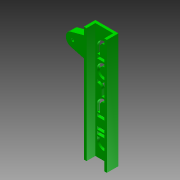
# Autodesk Inventor part: TabletMount-Mast-Left
Saved by Autodesk Inventor 2012 (Build 160160000, 160)
## iProperties
Created: 2013-10-06
Part Number: TabletMount-Mast-Left
Material: Default
Document SubType Name: Modeling
Designer: joe_000
Density: 1 g/cm^3
Author: joe_000
Autodesk Inventor part; units mm, degrees
ref_plane "YZ Plane" through (0, 0, 0) normal (1, 0, 0) x (0, 1, 0)
ref_plane "XZ Plane" through (0, 0, 0) normal (0, 1, 0) x (-1, 0, 0)
ref_plane "XY Plane" through (0, 0, 0) normal (0, 0, 1) x (1, 0, 0)
sketch "Sketch1" plane through (0, 0, 0) normal (0, 1, 0) x (-1, 0, 0)
  line L0 (0, 12.7) -> (0, 0)
  line L1 (0, 0) -> (25.4, 0)
  line L2 (25.4, 0) -> (25.4, 12.7)
  line L3 (25.4, 12.7) -> (22.479, 12.7)
  line L4 (22.479, 12.7) -> (22.479, 2.921)
  line L5 (22.479, 2.921) -> (2.921, 2.921)
  line L6 (2.921, 2.921) -> (2.921, 12.7)
  line L7 (2.921, 12.7) -> (0, 12.7)
  dimension "d0" = 19.558
  dimension "d1" = 2.921
  dimension "d2" = 2.921
  dimension "d3" = 2.921
  dimension "d4" = 9.779
  constraints: 16 end point, 5 parallel, 1 collinear, 1 horizontal, 1 perpendicular, 1 vertical
  measures "d0" distance of L4.end L5.end
  measures "d1" distance between parallel lines of L0 L6
  measures "d2" distance between parallel lines of L2 L4
  measures "d3" distance between parallel lines of L1 L5
  measures "d4" distance between parallel lines of L5 L3
extrude "Extrusion1" add sketch "Sketch1" along normal blind 127
sketch "Sketch3" plane through (0, 0, 0) normal (0, 0, -1) x (-1, 0, 0)
  line L0 (0, 0) -> (0, 127) projected
  line L1 (25.4, 0) -> (25.4, 127) projected
  line L2 (25.4, 115.4147) -> (44.45, 110.3102)
  line L3 (25.4, 90.8361) -> (44.45, 95.9406)
  arc A0 (44.45, 95.9406) -> (44.45, 110.3102) centre (42.5248, 103.1254) ccw
  point P0 (0, 115.8525)
  point P1 (0, 86.0657)
  dimension "d9" = 75
  dimension "d10" = 75
  dimension "d11" = 19.05
  dimension "d12" = 19.05
  constraints: 4 end point, 4 point on line, 2 point on circle, 1 centre point, 1 tangent
  measures "d9" angle of L1 L2
  measures "d10" angle of L1 L3
  measures "d11" horizontal distance of L2.start L2.end
  measures "d12" horizontal distance of L3.start L3.end
extrude "Extrusion2" add sketch "Sketch3" against normal blind 8.0433
hole "Hole1" at (-42.5248, 103.1254, 0) direction (0, 0, 1) diameter 3 end through all
fillet "Fillet1" radius 3.175 2 edges at (-25.4, 115.4147, 4.0217) (-25.4, 90.8361, 4.0217)
sketch "Sketch4" plane through (0, 0, 0) normal (0, 0, -1) x (-1, 0, 0)
  line L0 (5.2487, 9.5266) -> (5.2487, 115.9417) construction
  line L1 (5.2487, 115.9417) -> (20.5107, 115.9417) construction
  line L2 (20.5107, 115.9417) -> (20.5107, 9.5266) construction
  line L3 (20.5107, 9.5266) -> (5.2487, 9.5266) construction
  line L4 (5.2487, 17.8252) -> (5.2487, 24.8769)
  line L5 (5.2487, 24.8769) -> (20.5107, 24.8769)
  line L6 (20.5107, 24.8769) -> (20.5107, 21.8201)
  line L7 (20.5107, 21.8201) -> (8.2172, 21.8201)
  line L8 (8.2172, 21.8201) -> (8.2283, 19.0833)
  line L9 (8.2283, 19.0833) -> (8.2283, 18.4322)
  spline S0 degree 2 poles (8.2283, 18.4322) (8.2283, 16.1479) (8.4159, 15.894) knots 0 0 0 1 1 1
  spline S1 degree 2 poles (8.4159, 15.894) (8.7911, 14.5256) (9.9939, 13.5766) knots 0 0 0 1 1 1
  spline S2 degree 2 poles (9.9939, 13.5766) (11.4506, 12.5613) (12.8852, 12.5613) knots 0 0 0 1 1 1
  spline S3 degree 2 poles (12.8852, 12.5613) (14.673, 12.5613) (16.1628, 13.9408) knots 0 0 0 1 1 1
  spline S4 degree 2 poles (16.1628, 13.9408) (17.0346, 14.8677) (17.2222, 15.5299) knots 0 0 0 1 1 1
  spline S5 degree 2 poles (17.2222, 15.5299) (17.5532, 16.192) (17.5532, 17.8252) knots 0 0 0 1 1 1
  line L10 (17.5532, 17.8252) -> (17.5532, 19.9551)
  line L11 (17.5532, 19.9551) -> (20.5107, 19.9551)
  line L12 (20.5107, 19.9551) -> (20.5107, 17.4059)
  spline S6 degree 2 poles (20.5107, 17.4059) (20.5107, 14.5698) (19.021, 12.6055) knots 0 0 0 1 1 1
  spline S7 degree 2 poles (19.021, 12.6055) (17.8953, 11.1929) (16.9904, 10.7074) knots 0 0 0 1 1 1
  spline S8 degree 2 poles (16.9904, 10.7074) (15.1034, 9.5266) (13.128, 9.5266) knots 0 0 0 1 1 1
  line L13 (13.128, 9.5266) -> (12.6866, 9.5266)
  spline S9 degree 2 poles (12.6866, 9.5266) (9.9388, 9.5266) (7.6323, 11.5902) knots 0 0 0 1 1 1
  spline S10 degree 2 poles (7.6323, 11.5902) (6.4184, 12.8372) (6.0984, 13.6318) knots 0 0 0 1 1 1
  spline S11 degree 2 poles (6.0984, 13.6318) (5.7894, 14.2056) (5.5025, 15.2098) knots 0 0 0 1 1 1
  spline S12 degree 2 poles (5.5025, 15.2098) (5.2487, 16.1147) (5.2487, 17.8252) knots 0 0 0 1 1 1
  spline S13 degree 2 poles (5.2707, 34.1578) (5.2707, 37.8215) (8.2945, 40.2935) knots 0 0 0 1 1 1
  spline S14 degree 2 poles (8.2945, 40.2935) (8.9125, 40.7459) (9.3428, 40.9556) knots 0 0 0 1 1 1
  spline S15 degree 2 poles (9.3428, 40.9556) (9.8615, 41.2425) (10.7443, 41.5074) knots 0 0 0 1 1 1
  spline S16 degree 2 poles (10.7443, 41.5074) (11.8038, 41.8274) (13.6246, 41.8274) knots 0 0 0 1 1 1
  line L14 (13.6246, 41.8274) -> (20.5107, 41.8274)
  line L15 (20.5107, 41.8274) -> (20.5107, 38.7706)
  line L16 (20.5107, 38.7706) -> (13.2935, 38.7706)
  spline S17 degree 2 poles (13.2935, 38.7706) (9.6518, 38.7706) (8.4159, 35.482) knots 0 0 0 1 1 1
  spline S18 degree 2 poles (8.4159, 35.482) (8.2062, 34.7206) (8.1951, 34.1578) knots 0 0 0 1 1 1
  spline S19 degree 2 poles (8.1951, 34.1578) (8.2062, 33.5839) (8.4159, 32.8445) knots 0 0 0 1 1 1
  spline S20 degree 2 poles (8.4159, 32.8445) (9.6518, 29.5449) (13.2935, 29.5449) knots 0 0 0 1 1 1
  line L17 (13.2935, 29.5449) -> (20.5107, 29.5449)
  line L18 (20.5107, 29.5449) -> (20.5107, 26.4771)
  line L19 (20.5107, 26.4771) -> (13.6246, 26.4771)
  spline S21 degree 2 poles (13.6246, 26.4771) (11.8038, 26.4771) (10.7443, 26.7971) knots 0 0 0 1 1 1
  spline S22 degree 2 poles (10.7443, 26.7971) (9.8615, 27.0619) (9.3428, 27.3599) knots 0 0 0 1 1 1
  spline S23 degree 2 poles (9.3428, 27.3599) (8.9014, 27.5585) (8.2945, 28.022) knots 0 0 0 1 1 1
  spline S24 degree 2 poles (8.2945, 28.022) (5.2707, 30.494) (5.2707, 34.1578) knots 0 0 0 1 1 1
  spline S25 degree 2 poles (5.2597, 48.8901) (5.2597, 51.969) (5.3921, 52.4325) knots 0 0 0 1 1 1
  spline S26 degree 2 poles (5.3921, 52.4325) (5.5356, 53.6795) (6.4405, 55.2466) knots 0 0 0 1 1 1
  spline S27 degree 2 poles (6.4405, 55.2466) (6.9702, 56.0963) (8.0627, 57.0674) knots 0 0 0 1 1 1
  spline S28 degree 2 poles (8.0627, 57.0674) (10.1926, 58.7779) (12.8963, 58.7779) knots 0 0 0 1 1 1
  spline S29 degree 2 poles (12.8963, 58.7779) (14.4854, 58.7779) (15.8979, 58.171) knots 0 0 0 1 1 1
  spline S30 degree 2 poles (15.8979, 58.171) (18.6347, 56.9571) (19.8597, 54.1982) knots 0 0 0 1 1 1
  spline S31 degree 2 poles (19.8597, 54.1982) (20.5107, 52.9181) (20.5107, 50.2585) knots 0 0 0 1 1 1
  line L20 (20.5107, 50.2585) -> (20.5107, 43.7697)
  line L21 (20.5107, 43.7697) -> (20.4445, 43.4276)
  line L22 (20.4445, 43.4276) -> (17.5532, 43.4276)
  line L23 (17.5532, 43.4276) -> (17.5532, 50.5896)
  spline S32 degree 2 poles (17.5532, 50.5896) (17.5532, 51.7262) (17.3436, 52.3553) knots 0 0 0 1 1 1
  spline S33 degree 2 poles (17.3436, 52.3553) (16.7808, 54.0106) (15.6772, 54.7941) knots 0 0 0 1 1 1
  spline S34 degree 2 poles (15.6772, 54.7941) (14.2647, 55.7321) (12.9294, 55.7321) knots 0 0 0 1 1 1
  spline S35 degree 2 poles (12.9294, 55.7321) (11.583, 55.7321) (10.2809, 54.9155) knots 0 0 0 1 1 1
  spline S36 degree 2 poles (10.2809, 54.9155) (9.5304, 54.4079) (9.1442, 53.7899) knots 0 0 0 1 1 1
  spline S37 degree 2 poles (9.1442, 53.7899) (8.2172, 52.6753) (8.2172, 50.5896) knots 0 0 0 1 1 1
  line L24 (8.2172, 50.5896) -> (8.2172, 43.4276)
  line L25 (8.2172, 43.4276) -> (5.2597, 43.4276)
  line L26 (5.2597, 43.4276) -> (5.2597, 48.8901)
  line L27 (5.2597, 60.3781) -> (5.2597, 70.1776)
  spline S38 degree 2 poles (5.2597, 70.1776) (5.2597, 72.7819) (6.8157, 74.2497) knots 0 0 0 1 1 1
  spline S39 degree 2 poles (6.8157, 74.2497) (7.4227, 74.9008) (7.9965, 75.1546) knots 0 0 0 1 1 1
  spline S40 degree 2 poles (7.9965, 75.1546) (9.1442, 75.7284) (10.2367, 75.7284) knots 0 0 0 1 1 1
  line L28 (10.2367, 75.7284) -> (10.6671, 75.7284)
  spline S41 degree 2 poles (10.6671, 75.7284) (12.3335, 75.7284) (13.9336, 74.2828) knots 0 0 0 1 1 1
  spline S42 degree 2 poles (13.9336, 74.2828) (14.8275, 73.3448) (15.0813, 72.5833) knots 0 0 0 1 1 1
  spline S43 degree 2 poles (15.0813, 72.5833) (17.1339, 74.5145) (20.5107, 74.5145) knots 0 0 0 1 1 1
  line L29 (20.5107, 74.5145) -> (20.5107, 71.4356)
  line L30 (20.5107, 71.4356) -> (20.279, 71.4356)
  spline S44 degree 2 poles (20.279, 71.4356) (17.785, 71.4356) (16.3062, 69.4051) knots 0 0 0 1 1 1
  spline S45 degree 2 poles (16.3062, 69.4051) (15.4896, 68.2574) (15.4896, 66.3924) knots 0 0 0 1 1 1
  line L31 (15.4896, 66.3924) -> (15.4896, 60.3781)
  line L32 (15.4896, 60.3781) -> (12.5542, 60.3781)
  line L33 (12.5542, 60.3781) -> (12.5542, 70.3762)
  spline S46 degree 2 poles (12.5542, 70.3762) (12.5542, 72.0095) (10.9319, 72.5943) knots 0 0 0 1 1 1
  spline S47 degree 2 poles (10.9319, 72.5943) (10.6009, 72.6606) (10.3802, 72.6826) knots 0 0 0 1 1 1
  spline S48 degree 2 poles (10.3802, 72.6826) (9.4753, 72.6826) (8.7469, 71.9322) knots 0 0 0 1 1 1
  spline S49 degree 2 poles (8.7469, 71.9322) (8.2393, 71.2811) (8.2393, 70.5528) knots 0 0 0 1 1 1
  spline S50 degree 2 poles (8.2393, 70.5528) (8.1951, 70.5528) (8.1951, 70.1114) knots 0 0 0 1 1 1
  line L34 (8.1951, 70.1114) -> (8.1951, 60.3781)
  line L35 (8.1951, 60.3781) -> (5.2597, 60.3781)
  line L36 (5.2707, 84.9651) -> (5.2707, 85.0644)
  spline S51 degree 2 poles (5.2707, 85.0644) (5.2707, 88.5848) (8.151, 91.0677) knots 0 0 0 1 1 1
  spline S52 degree 2 poles (8.151, 91.0677) (10.3029, 92.6789) (12.8521, 92.6789) knots 0 0 0 1 1 1
  line L37 (12.8521, 92.6789) -> (12.9514, 92.6789)
  spline S53 degree 2 poles (12.9514, 92.6789) (16.4718, 92.6789) (18.9216, 89.7435) knots 0 0 0 1 1 1
  spline S54 degree 2 poles (18.9216, 89.7435) (20.5107, 87.6026) (20.5107, 85.0424) knots 0 0 0 1 1 1
  line L38 (20.5107, 85.0424) -> (20.5107, 84.943)
  spline S55 degree 2 poles (20.5107, 84.943) (20.5107, 81.4448) (17.6526, 78.9618) knots 0 0 0 1 1 1
  spline S56 degree 2 poles (17.6526, 78.9618) (16.4387, 78.09) (15.4234, 77.7369) knots 0 0 0 1 1 1
  spline S57 degree 2 poles (15.4234, 77.7369) (14.1543, 77.3286) (12.9294, 77.3286) knots 0 0 0 1 1 1
  line L39 (12.9294, 77.3286) -> (12.8301, 77.3286)
  spline S58 degree 2 poles (12.8301, 77.3286) (9.3759, 77.3286) (6.915, 80.1757) knots 0 0 0 1 1 1
  spline S59 degree 2 poles (6.915, 80.1757) (5.5356, 82.1069) (5.3701, 83.696) knots 0 0 0 1 1 1
  spline S60 degree 2 poles (5.3701, 83.696) (5.2707, 84.1816) (5.2707, 84.9651) knots 0 0 0 1 1 1
  spline S61 degree 2 poles (12.8632, 80.3744) (14.8606, 80.3744) (16.3614, 81.9304) knots 0 0 0 1 1 1
  spline S62 degree 2 poles (16.3614, 81.9304) (17.5532, 83.3208) (17.5532, 84.8437) knots 0 0 0 1 1 1
  line L40 (17.5532, 84.8437) -> (17.5532, 85.1417)
  spline S63 degree 2 poles (17.5532, 85.1417) (17.5532, 86.3666) (16.7145, 87.6467) knots 0 0 0 1 1 1
  spline S64 degree 2 poles (16.7145, 87.6467) (15.7434, 88.96) (14.2536, 89.4235) knots 0 0 0 1 1 1
  spline S65 degree 2 poles (14.2536, 89.4235) (13.8674, 89.5669) (12.9073, 89.6331) knots 0 0 0 1 1 1
  spline S66 degree 2 poles (12.9073, 89.6331) (10.9651, 89.6331) (9.4642, 88.1213) knots 0 0 0 1 1 1
  spline S67 degree 2 poles (9.4642, 88.1213) (8.2062, 86.6977) (8.2062, 85.0093) knots 0 0 0 1 1 1
  spline S68 degree 2 poles (8.2062, 85.0093) (8.2062, 83.0229) (9.8615, 81.4889) knots 0 0 0 1 1 1
  spline S69 degree 2 poles (9.8615, 81.4889) (10.7112, 80.8489) (11.2961, 80.6723) knots 0 0 0 1 1 1
  spline S70 degree 2 poles (11.2961, 80.6723) (12.1238, 80.3744) (12.8632, 80.3744) knots 0 0 0 1 1 1
  line L41 (5.2707, 94.2791) -> (5.2707, 97.3359)
  line L42 (5.2707, 97.3359) -> (20.5107, 97.3359)
  line L43 (20.5107, 97.3359) -> (20.5107, 94.2791)
  line L44 (20.5107, 94.2791) -> (5.2707, 94.2791)
  spline S71 degree 2 poles (5.2597, 104.4538) (5.2597, 107.5327) (5.3921, 107.9962) knots 0 0 0 1 1 1
  spline S72 degree 2 poles (5.3921, 107.9962) (5.5356, 109.2432) (6.4405, 110.8102) knots 0 0 0 1 1 1
  spline S73 degree 2 poles (6.4405, 110.8102) (6.9702, 111.6599) (8.0627, 112.6311) knots 0 0 0 1 1 1
  spline S74 degree 2 poles (8.0627, 112.6311) (10.1926, 114.3416) (12.8963, 114.3416) knots 0 0 0 1 1 1
  spline S75 degree 2 poles (12.8963, 114.3416) (14.4854, 114.3416) (15.8979, 113.7346) knots 0 0 0 1 1 1
  spline S76 degree 2 poles (15.8979, 113.7346) (18.6347, 112.5207) (19.8597, 109.7618) knots 0 0 0 1 1 1
  spline S77 degree 2 poles (19.8597, 109.7618) (20.5107, 108.4817) (20.5107, 105.8222) knots 0 0 0 1 1 1
  line L45 (20.5107, 105.8222) -> (20.5107, 99.3333)
  line L46 (20.5107, 99.3333) -> (20.4445, 98.9912)
  line L47 (20.4445, 98.9912) -> (17.5532, 98.9912)
  line L48 (17.5532, 98.9912) -> (17.5532, 106.1532)
  spline S78 degree 2 poles (17.5532, 106.1532) (17.5532, 107.2899) (17.3436, 107.9189) knots 0 0 0 1 1 1
  spline S79 degree 2 poles (17.3436, 107.9189) (16.7808, 109.5742) (15.6772, 110.3578) knots 0 0 0 1 1 1
  spline S80 degree 2 poles (15.6772, 110.3578) (14.2647, 111.2958) (12.9294, 111.2958) knots 0 0 0 1 1 1
  spline S81 degree 2 poles (12.9294, 111.2958) (11.583, 111.2958) (10.2809, 110.4792) knots 0 0 0 1 1 1
  spline S82 degree 2 poles (10.2809, 110.4792) (9.5304, 109.9715) (9.1442, 109.3535) knots 0 0 0 1 1 1
  spline S83 degree 2 poles (9.1442, 109.3535) (8.2172, 108.239) (8.2172, 106.1532) knots 0 0 0 1 1 1
  line L49 (8.2172, 106.1532) -> (8.2172, 98.9912)
  line L50 (8.2172, 98.9912) -> (5.2597, 98.9912)
  line L51 (5.2597, 98.9912) -> (5.2597, 104.4538)
  constraints: 2 other
extrude "Extrusion3" cut sketch "Sketch4" against normal up to next
sketch "Sketch6" plane through (0, 0, 0) normal (0, 0, -1) x (-1, 0, 0)
  line L0 (24.3591, 83.9985) -> (4.1153, 83.9985)
  line L1 (4.1153, 83.9985) -> (4.1153, 85.2685)
  line L2 (4.1153, 85.2685) -> (24.3591, 85.2685)
  line L3 (24.3591, 85.2685) -> (24.3591, 83.9985)
  dimension "d25" = 1.27
  constraints: 8 end point, 2 parallel, 1 horizontal, 1 perpendicular
  measures "d25" distance of L0.end L1.end
extrude "Extrusion5" add sketch "Sketch6" against normal blind 1.27
equation "\"d0\" = MastWidth + 2 * MastTolerance"
equation "\"d1\" = WallThickness"
equation "\"d2\" = WallThickness"
equation "\"d3\" = WallThickness"
equation "\"d4\" = 0.5 * MastWidth + MastTolerance"
equation "\"d5\" = Length"
equation "\"d9\" = HingeAngle"
equation "\"d10\" = HingeAngle"
equation "\"d11\" = HingeLength"
equation "\"d12\" = HingeLength"
equation "\"d13\" = HingeHoleDiameter"
equation "\"MastWidth\" = 19.05"
equation "\"MastTolerance\" = 0.254"
equation "\"WallThickness\" = 2.921"
equation "\"Length\" = 127"
equation "\"HingeAngle\" = 75deg"
equation "\"HingeLength\" = 19.05"
equation "\"HingeHoleDiameter\" = 3"
body "Solid1"
